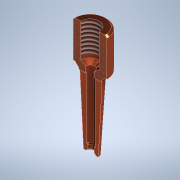
# Autodesk Inventor part: FilamentPin
Saved by Autodesk Inventor 2022 (Build 260153000, 153)
## iProperties
Created: 2021-11-15
Part Number: FilamentPin
Material: Copper
Document SubType Name: Modeling
Designer: vinicius.miguel
Density: 8.94 g/cm^3
Appearance: Copper - Polished
Mass: 0.638403 g
Surface Area: 2.2529 cm^2
Volume: 0.0714097 cm^3
Author: vinicius.miguel
Autodesk Inventor part; units mm, degrees
ref_plane "YZ Plane" through (0, 0, 0) normal (1, 0, 0) x (0, 1, 0)
ref_plane "XZ Plane" through (0, 0, 0) normal (0, 1, 0) x (-1, 0, 0)
ref_plane "XY Plane" through (0, 0, 0) normal (0, 0, 1) x (1, 0, 0)
sketch "Sketch1" plane through (0, 0, 0) normal (0, 0, 1) x (1, 0, 0)
  line L0 (0, 0) -> (0, -5.8)
  line L1 (0, 0) -> (2.25, 0)
  line L2 (2.25, 0) -> (2.25, -5)
  line L3 (2.25, -5) -> (1.5, -5)
  line L4 (1.5, -5) -> (1.5, -14.7)
  line L5 (1.5, -14.7) -> (0.7, -14.7)
  line L6 (0.7, -14.7) -> (0.45, -14.45)
  line L7 (0.45, -14.45) -> (0.45, -13.95)
  line L8 (0.45, -13.95) -> (0.6, -13.8)
  line L9 (0.6, -13.8) -> (0.6, -5.8)
  line L10 (0.6, -5.8) -> (0, -5.8)
  line L11 (1, -14.7) -> (1.5, -5.5)
  line L12 (0.6, -5.8) -> (0.6, 0)
  dimension "d0" = 4.5
  dimension "d1" = 0.9
  dimension "d2" = 1.2
  dimension "d3" = 135
  dimension "d4" = 3
  dimension "d5" = 5
  dimension "d6" = 0.8
  dimension "d7" = 8
  dimension "d8" = 0.25
  dimension "d9" = 0.5
  dimension "d10" = 0.5
  dimension "d11" = 0.3
  constraints: 26 end point, 7 perpendicular, 3 point on line, 2 parallel, 1 horizontal, 1 vertical
  measures "d0" diameter of L2 L0
  measures "d1" diameter of L7 L0
  measures "d2" diameter of L9 L0
  measures "d3" angle of L9 L8
  measures "d4" diameter of L4 L0
  measures "d5" distance of L1.end L2.end
  measures "d6" distance between parallel lines of L3 L10
  measures "d7" distance of L8.end L9.end
  measures "d8" distance from line of L5.end L7
  measures "d9" distance of L6.end L7.end
  measures "d10" distance of L3.end L11.end
  measures "d11" distance of L11.start L5.end
revolve "Revolution1" add sketch "Sketch1" angle 360 about axis through (0, 0, 0) along (0, -1, 0) contours L1 L2 L3 L4 L11 L5 L6 L7 L8 L9 L12
sketch "Sketch3" plane through (0, 0, 0) normal (0, 1, 0) x (1, 0, 0)
  circle A0 centre (0, 0) radius 0.6 projected
  constraints: 1 coincident
hole "Hole1" at (0, 0, 0) direction (0, -1, 0) diameter 2.459 depth 4.5 tip angle 118 thread size "M3x0.5" class "6H" standard "ISO Metric profile"
chamfer "Chamfer2" distance 0.25 angle 45 1 edges at (-2.25, 0, 0)
sketch "Sketch2" plane through (0, -14.7, 0) normal (0, -1, 0) x (1, 0, 0)
  line L0 (-0.125, -2.2191) -> (0.125, -2.2191)
  line L1 (0.125, -2.2191) -> (0.125, 2.2191)
  line L2 (0.125, 2.2191) -> (-0.125, 2.2191)
  line L3 (-0.125, 2.2191) -> (-0.125, -2.2191)
  line L4 (-0.125, -2.2191) -> (0.125, 2.2191) construction
  line L5 (0.125, -2.2191) -> (-0.125, 2.2191) construction
  line L6 (-2.0682, -0.125) -> (2.0682, -0.125)
  line L7 (2.0682, -0.125) -> (2.0682, 0.125)
  line L8 (2.0682, 0.125) -> (-2.0682, 0.125)
  line L9 (-2.0682, 0.125) -> (-2.0682, -0.125)
  line L10 (-2.0682, -0.125) -> (2.0682, 0.125) construction
  line L11 (2.0682, -0.125) -> (-2.0682, 0.125) construction
  point P0 (0, 0)
  point P1 (-0.125, -0.125)
  point P2 (0.125, -0.125)
  point P3 (0.125, 0.125)
  point P4 (-0.125, 0.125)
  dimension "d13" = 0.25
  dimension "d14" = 0.25
  constraints: 24 end point, 4 midpoint, 4 parallel, 2 horizontal, 2 perpendicular
  measures "d13" distance of L6.end L7.end
  measures "d14" distance of L0.start L0.end
extrude "Extrusion1" cut sketch "Sketch2" against normal blind 9
chamfer "Chamfer3" distance 0.5 angle 45 1 edges at (-1.5, -5, 0)
equation "\"d13\" = d14"
body "Solid1"
